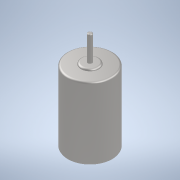
# Autodesk Inventor part: Motor DC
Saved by Autodesk Inventor 2020.1 (Build 241239000, 239)
## iProperties
Created: 2020-03-26
Part Number: Motor DC
Material: Stainless Steel, Brushed
Document SubType Name: Modeling
Designer: Daniel
Density: 8 g/cm^3
Appearance: Stainless - Brushed
Author: Daniel
Autodesk Inventor part; units mm, degrees
ref_plane "YZ Plane" through (0, 0, 0) normal (1, 0, 0) x (0, 1, 0)
ref_plane "XZ Plane" through (0, 0, 0) normal (0, 1, 0) x (-1, 0, 0)
ref_plane "XY Plane" through (0, 0, 0) normal (0, 0, 1) x (1, 0, 0)
sketch "Sketch1" plane through (0, 0, 0) normal (0, 1, 0) x (-1, 0, 0)
  circle A0 centre (0, 0) radius 25
  dimension "d0" = 50
  constraints: 1 centre point, 1 coincident
  measures "d0" diameter of A0
extrude "Extrusion1" add sketch "Sketch1" along normal blind 80
sketch "Sketch2" plane through (0, 80, 0) normal (0, 1, 0) x (1, 0, 0)
  circle A0 centre (0, 0) radius 10
  circle A1 centre (0, 0) radius 2.5
  dimension "d3" = 20
  dimension "d4" = 5
  constraints: 2 centre point, 2 coincident
  measures "d3" diameter of A0
  measures "d4" diameter of A1
extrude "Extrusion2" add sketch "Sketch2" along normal blind 2 contours A0 | A1
extrude "Extrusion3" add sketch "Sketch2" along normal blind 30 contours A1
fillet "Fillet1" radius 2 3 edges at (25, 0, 0) (25, 80, 0) (-10, 82, 0)
fillet "Fillet2" radius 1 1 edges at (-2.5, 110, 0)
body "Solid1"
